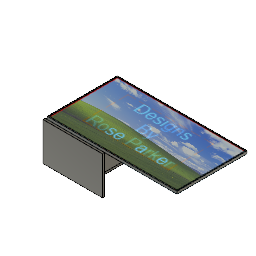
Designs by Rose Parker v1 (Autodesk Fusion 360 design; units mm, degrees)
Autodesk Fusion 360 part; units mm, degrees
sketch "Sketch1" plane through (0, 0, 0) normal (0, 0, 1) x (1, 0, 0)
  line L0 (-30, 15) -> (31, 15)
  line L1 (31, 15) -> (31, -18)
  line L2 (31, -18) -> (-30, -18)
  line L3 (-30, -18) -> (-30, 15)
  line L4 (-29.48, 14.4823) -> (30.5108, 14.4823)
  line L5 (30.5108, 14.4823) -> (30.5108, -17.4715)
  line L6 (30.5108, -17.4715) -> (-29.48, -17.4715)
  line L7 (-29.48, -17.4715) -> (-29.48, 14.4823)
  constraint horizontal L0
  constraint vertical L1
  constraint horizontal L2
  constraint vertical L3
  constraint horizontal L4
  constraint vertical L5
  constraint horizontal L6
  constraint vertical L7
extrude "Extrude1" add sketch "Sketch1" along normal blind 1.3
sketch "Sketch2" plane through (0, 0, 0) normal (0, 0, 1) x (1, 0, 0)
  line L0 (30.5108, -17.4715) -> (-29.48, -17.4715)
  line L1 (-29.48, -17.4715) -> (-29.48, 14.4823)
  line L2 (-29.48, 14.4823) -> (30.5108, 14.4823)
  line L3 (30.5108, 14.4823) -> (30.5108, -17.4715)
  point P0 (30.5108, -17.4715)
  point P1 (-29.48, 14.4823)
  constraint horizontal L0
  constraint vertical L1
  constraint horizontal L2
  constraint vertical L3
  constraint coincident P1 L1.end
  constraint coincident P0 L0.start
extrude "Extrude2" add sketch "Sketch2" along normal blind 1
sketch "Sketch3" plane through (0, 0, 0) normal (0, 0, -1) x (1, 0, 0)
  line L0 (31, 18) -> (-30, 18)
  line L1 (-30, 18) -> (-30, -15)
  line L2 (-30, -15) -> (31, -15)
  line L3 (31, -15) -> (31, 18)
  line L4 (5, -5) -> (-5, -5)
  line L5 (-5, -5) -> (-5, 35)
  line L6 (-5, 35) -> (5, 35)
  line L7 (5, 35) -> (5, -5)
  constraint horizontal L4
  constraint vertical L5
  constraint horizontal L6
  constraint vertical L7
extrude "Extrude3" add sketch "Sketch3" along normal blind 1 contours L0 L4 L5 L7 | L0 L5 L6 L7
sketch "Sketch4" plane through (0, 0, 0) normal (0, 0, -1) x (1, 0, 0)
  line L0 (-5, -5) -> (-5, 18)
  line L1 (-5, 18) -> (-30, 18)
  line L2 (-30, 18) -> (-30, -15)
  line L3 (-30, -15) -> (31, -15)
  line L4 (31, -15) -> (31, 18)
  line L5 (31, 18) -> (5, 18)
  line L6 (5, 18) -> (5, -5)
  line L7 (5, -5) -> (-5, -5)
sketch "Sketch5" plane through (0, 0, 0) normal (0, 1, 0) x (1, 0, 0)
sketch "Sketch6" plane through (0, 0, 1) normal (0, 0, 1) x (-1, 0, 0)
  line L0 (-30.5108, -14.4823) -> (29.48, -14.4823)
  line L1 (29.48, -14.4823) -> (29.48, 17.4715)
  line L2 (29.48, 17.4715) -> (-30.5108, 17.4715)
  line L3 (-30.5108, 17.4715) -> (-30.5108, -14.4823)
  line L4 (20, 11) -> (-20, 11) construction
  line L5 (-20, 11) -> (-20, -10) construction
  line L6 (-20, -10) -> (20, -10) construction
  line L7 (20, -10) -> (20, 11) construction
  dimension "d7" = 5
sketch "Sketch7" plane through (0, 0, 0) normal (1, 0, 0) x (0, 1, 0)
sketch "Sketch8" plane through (0, 0, 0) normal (0, 0, 1) x (1, 0, 0)
  line L0 (-14, -35) -> (13, -35)
  line L1 (13, -35) -> (13, -36)
  line L2 (13, -36) -> (-14, -36)
  line L3 (-14, -36) -> (-14, -35)
  constraint horizontal L0
  constraint vertical L1
  constraint horizontal L2
  constraint vertical L3
extrude "Extrude4" add sketch "Sketch8" along normal blind 17
extrude "Extrude5" add 1 faces at (-2, -35.6667, 0) along direction (0, 0, -1) blind 1
extrude "Extrude6" add 1 faces at (13, -35.3333, 11) along direction (1, 0, 0) blind 1
